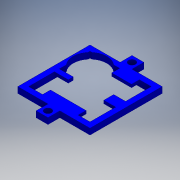
# Autodesk Inventor part: MCP73871_holder
Saved by Autodesk Inventor 2018 (Build 220112000, 112)
## iProperties
Created: 2019-09-05
Part Number: MCP73871_holder
Material: Generic
Document SubType Name: Modeling
Designer: ZEUSLAP
Density: 1 g/cm^3
Appearance: Default
Author: ZEUSLAP
## iProperties of the stored document MCP73871_holder_3DPrint.ipt
Created: 2019-09-05
Part Number: MCP73871_holder_3DPrint
Material: Generic
Document SubType Name: Modeling
Designer: ZEUSLAP
Density: 1 g/cm^3
Appearance: Default
Author: ZEUSLAP
Autodesk Inventor part; units mm, degrees
ref_plane "YZ Plane" through (0, 0, 0) normal (1, 0, 0) x (0, 1, 0)
ref_plane "XZ Plane" through (0, 0, 0) normal (0, 1, 0) x (-1, 0, 0)
ref_plane "XY Plane" through (0, 0, 0) normal (0, 0, 1) x (1, 0, 0)
sketch "shape" plane through (0, 0, 0) normal (0, 0, 1) x (1, 0, 0)
  line L0 (-18.25, 18.25) -> (18.25, 18.25)
  line L1 (18.25, 18.25) -> (18.25, -18.25)
  line L2 (18.25, -18.25) -> (-18.25, -18.25)
  line L3 (-18.25, -18.25) -> (-18.25, 18.25)
  line L4 (-15.5, 15.5) -> (15.5, 15.5)
  line L5 (15.5, 15.5) -> (15.5, -15.5)
  line L6 (15.5, -15.5) -> (-15.5, -15.5)
  line L7 (-15.5, -15.5) -> (-15.5, 15.5)
  line L8 (9.5, 2.5) -> (15.5, 2.5)
  line L9 (15.5, 2.5) -> (15.5, -2.5)
  line L10 (15.5, -2.5) -> (9.5, -2.5)
  line L11 (9.5, -2.5) -> (9.5, 2.5)
  line L12 (-0.5, 15.5) -> (9.5, 15.5)
  line L13 (9.5, 15.5) -> (9.5, 11.5)
  line L14 (9.5, 11.5) -> (-0.5, 11.5)
  line L15 (-0.5, 11.5) -> (-0.5, 15.5)
  line L16 (-8.5, -11.5) -> (9.5, -11.5)
  line L17 (9.5, -11.5) -> (9.5, -15.5)
  line L18 (9.5, -15.5) -> (-8.5, -15.5)
  line L19 (-8.5, -15.5) -> (-8.5, -11.5)
  line L20 (-15.5, 0) -> (-8.5, 0)
  line L21 (-8.5, 0) -> (-8.5, -2.5)
  line L22 (-8.5, -2.5) -> (-15.5, -2.5)
  line L23 (-15.5, -2.5) -> (-15.5, 0)
  circle A0 centre (-9, 9) radius 8.5
  line L24 (-3, 24.25) -> (3, 24.25)
  line L25 (3, 24.25) -> (3, 18.25)
  line L26 (3, 18.25) -> (-3, 18.25)
  line L27 (-3, 18.25) -> (-3, 24.25)
  line L28 (-3, -18.25) -> (3, -18.25)
  line L29 (3, -18.25) -> (3, -24.25)
  line L30 (3, -24.25) -> (-3, -24.25)
  line L31 (-3, -24.25) -> (-3, -18.25)
  circle A1 centre (0, -21.25) radius 1.75
  circle A2 centre (0, 21.25) radius 1.75
  point P0 (0, 0)
  point P1 (-18.25, 0)
  point P2 (0, 18.25)
  point P3 (-15.5, 0)
  point P4 (0, 15.5)
  point P5 (0, 24.25)
  point P6 (3, 21.25)
  point P7 (0, -24.25)
  point P8 (3, -21.25)
  dimension "d1" = 36.5
  dimension "d2" = 31
  dimension "d3" = 31
  dimension "d4" = 5
  dimension "d5" = 6
  dimension "d6" = 13
  dimension "d7" = 10
  dimension "d8" = 4
  dimension "d9" = 6
  dimension "d10" = 18
  dimension "d11" = 4
  dimension "d12" = 6
  dimension "d13" = 7
  dimension "d14" = 2.5
  dimension "d15" = 13
  dimension "d16" = 17
  dimension "d17" = 6.5
  dimension "d18" = 6.5
  dimension "d21" = 6
  dimension "d23" = 3.5
  constraints: 64 end point, 16 parallel, 8 horizontal, 8 midpoint, 8 perpendicular, 7 collinear, 5 vertical alignment, 4 equal length, 4 horizontal alignment, 3 centre point, 1 equal radius
  measures "d1" distance of L0.end L1.end
  measures "d2" distance of L5.end L6.end
  measures "d3" distance of L4.end L5.end
  measures "d4" distance of L10.end L8.start
  measures "d5" distance of L8.start L8.end
  measures "d6" distance between parallel lines of L6 L10
  measures "d7" distance of L13.end L14.end
  measures "d8" distance of L12.end L13.end
  measures "d9" distance between parallel lines of L5 L13
  measures "d10" distance of L16.start L16.end
  measures "d11" distance of L16.end L17.end
  measures "d12" distance between parallel lines of L5 L17
  measures "d13" distance of L21.end L22.end
  measures "d14" distance of L20.end L21.end
  measures "d15" distance between parallel lines of L22 L6
  measures "d16" diameter of A0
  measures "d17" distance from line of L7 A0.centre
  measures "d18" distance from line of L4 A0.centre
  measures "d21" distance of L28.end L29.end
  measures "d23" diameter of A1
extrude "over pcb" add sketch "shape" along normal blind 1.5 contours L0 L1 L2 L3 | L27 L24 L25 L0 | L2 L29 L30 L31 | L4 L13 L14 L15 | L5 L10 L11 L8 | L20 L21 L22 L7 | L6 L19 L16 L17
extrude "around pcb" add sketch "shape" against normal blind 1.5
equation "\"d18\" = d17"
body "Solid1"
